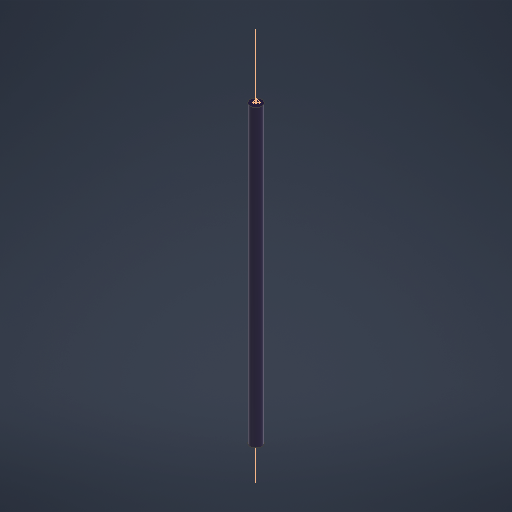
# Autodesk Inventor part: LOOP3_COLL_L
Saved by Autodesk Inventor 2026.1 (Build 301233000, 233)
## iProperties
Created: 2024-08-12
Part Number: LOOP3_COLL_L
Material: Generic
Document SubType Name: Modeling
Designer: User
Density: 1 g/cm^3
Appearance: Default
Author: User
Autodesk Inventor part; units mm, degrees
ref_plane "YZ Plane" through (0, 0, 0) normal (1, 0, 0) x (0, 1, 0)
ref_plane "XZ Plane" through (0, 0, 0) normal (0, 1, 0) x (-1, 0, 0)
ref_plane "XY Plane" through (0, 0, 0) normal (0, 0, 1) x (1, 0, 0)
sketch "Sketch1" plane through (0, 0, 0) normal (0, 1, 0) x (-1, 0, 0)
  circle A0 centre (0, 0) radius 1
  dimension "d0" = 2
  constraints: 1 centre point, 1 coincident
  measures "d0" diameter of A0
extrude "Extrusion1" add sketch "Sketch1" along normal blind 55
move faces "Move1" translate (0, -2.5, 0) faces at (-0.5848, 55, -0.397)
move faces "Move2" translate (0, -0.002, 0) faces at (-0.2495, 52.5, 0.221)
move faces "Move3" translate (0, -1.862, 0) faces at (-0.2495, 52.498, 0.221)
move faces "Move4" translate (0, -0.636, 0) faces at (-0.2495, 50.636, 0.221)
body "Solid1"
